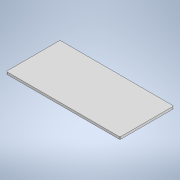
# Autodesk Inventor part: Internal Base Plate
Saved by Autodesk Inventor 2021 (Build 250183000, 183)
## iProperties
Created: 2020-07-02
Part Number: Internal Base Plate
Material: Generic
Document SubType Name: Modeling
Designer: jgray
Density: 1 g/cm^3
Appearance: Default
Author: jgray
Autodesk Inventor part; units mm, degrees
ref_plane "YZ Plane" through (0, 0, 0) normal (1, 0, 0) x (0, 1, 0)
ref_plane "XZ Plane" through (0, 0, 0) normal (0, 1, 0) x (-1, 0, 0)
ref_plane "XY Plane" through (0, 0, 0) normal (0, 0, 1) x (1, 0, 0)
sketch "Sketch1" plane through (0, 0, 0) normal (0, 1, 0) x (-1, 0, 0)
  line L0 (-121, 58.1) -> (121, 58.1)
  line L1 (123, 56.1) -> (123, -56.1)
  line L2 (121, -58.1) -> (-121, -58.1)
  line L3 (-123, -56.1) -> (-123, 56.1)
  line L4 (-123, 58.1) -> (123, -58.1) construction
  line L5 (123, 58.1) -> (-123, -58.1) construction
  arc A0 (121, -58.1) -> (123, -56.1) centre (121, -56.1) ccw
  arc A1 (123, 56.1) -> (121, 58.1) centre (121, 56.1) ccw
  arc A2 (-123, -56.1) -> (-121, -58.1) centre (-121, -56.1) ccw
  arc A3 (-121, 58.1) -> (-123, 56.1) centre (-121, 56.1) ccw
  point P0 (0, 0)
  dimension "d0" = 246
  dimension "d1" = 116.2
  dimension "d4" = 2
  constraints: 12 end point, 8 point on circle, 8 point on line, 8 tangent, 4 centre point, 3 equal radius, 2 midpoint, 2 parallel, 1 horizontal, 1 perpendicular
  measures "d0" distance of L4.end L5.end
  measures "d1" distance of L5.start L4.end
  measures "d4" radius of A0
extrude "Extrusion1" add sketch "Sketch1" along normal blind 5
body "Solid1"
